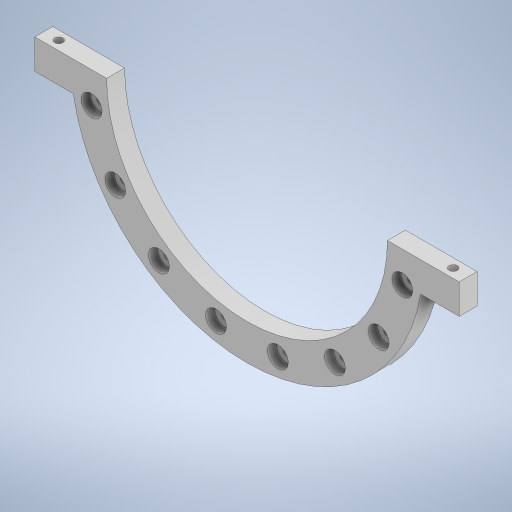
# Autodesk Inventor part: Постель 201 зад
Saved by Autodesk Inventor 2024.2 (Build 282272000, 272)
## iProperties
Created: 2024-04-28
Part Number: Постель 201 зад
Material: Generic
Document SubType Name: Sheet Metal
Designer: admin
Density: 1 g/cm^3
Appearance: Default
Stock Number: Постель_Корма
Flat Pattern Width: 29.5 cm
Flat Pattern Length: 71 cm
Flat Pattern Area: 2094.5 cm^2
Sheet Metal Rule: Default
Sheet Metal Width: 295,000 mm
Sheet Metal Length: 710,000 mm
Sheet Metal Area: 209450,000 mm^2
Author: pokla
Autodesk Inventor part; units mm, degrees
ref_plane "YZ Plane" through (0, 0, 0) normal (1, 0, 0) x (0, 1, 0)
ref_plane "XZ Plane" through (0, 0, 0) normal (0, 1, 0) x (-1, 0, 0)
ref_plane "XY Plane" through (0, 0, 0) normal (0, 0, 1) x (1, 0, 0)
sketch "Sketch1" plane through (0, 0, 0) normal (0, 0, 1) x (1, 0, 0)
  circle A0 centre (0, 0) radius 265 construction
  line L0 (0, 265) -> (0, 295) construction
  line L1 (0, 265) -> (0, 235) construction
  circle A1 centre (0, 0) radius 235
  circle A2 centre (0, 0) radius 295
  line L2 (-235, 0) -> (-235, 80) construction
  line L3 (-235, 80) -> (-295, 80) construction
  line L4 (-295, 80) -> (-295, 0) construction
  line L5 (235, 0) -> (235, 80) construction
  line L6 (235, 80) -> (295, 80) construction
  line L7 (295, 80) -> (295, 0) construction
  line L8 (-235, 0) -> (-295, 0)
  line L9 (-295, 0) -> (-355, 0)
  line L10 (-355, 0) -> (-355, -50)
  line L11 (-355, -50) -> (-290.7318, -50)
  line L12 (235, 0) -> (295, 0)
  line L13 (295, 0) -> (355, 0)
  line L14 (355, 0) -> (355, -50)
  line L15 (355, -50) -> (290.7318, -50)
  dimension "d13" = 530
  dimension "d26" = 80
  dimension "d36" = 60
  dimension "d40" = 60
  dimension "d41" = 50
  constraints: 32 end point, 8 point on circle, 7 perpendicular, 4 equal length, 4 horizontal, 4 tangent, 4 vertical, 3 coincident, 2 centre point, 1 line through centre, 1 point on line, 1 vertical alignment, 2 other
  measures "d26" distance of L2.start L2.end
  measures "d36" distance of L1.end L0.end
  measures "d40" distance of L4.end L9.end
  measures "d41" distance of L9.end L10.end
extrude "Extrusion1" add sketch "Sketch1" against normal blind 30 contours L12 A2 L8 A1 | L13 L14 L15 A2 | A2 L11 L10 L9 picked at (3.5144, -274.7637)
sketch "Sketch4" plane through (0, 0, 0) normal (0, 0, 1) x (1, 0, 0)
  line L0 (0, 0) -> (51.6989, -259.9081) construction
  line L1 (0, 0) -> (0, -276.8337) construction
  dimension "d27" = 265
  dimension "d35" = 11.25
  constraints: 4 end point, 1 coincident, 1 vertical
  measures "d27" distance of L0.end L0.start
  measures "d35" angle of L1 L0
sketch "Sketch7" plane through (0, 0, 0) normal (0, 0, 1) x (1, 0, 0)
  line L0 (-355, -50) -> (-355, 0) construction
  line L1 (-355, -25) -> (355, -25) construction
  line L2 (355, 0) -> (355, -50) construction
  point P0 (0, 0)
  point P1 (-330, -25)
  dimension "d42" = 25
  constraints: 2 end point, 2 midpoint, 1 point on line
  measures "d42" distance from line of point (-330, -25) L0
fillet "Fillet1" [suppressed]
hole "Hole1" [suppressed]
hole "Hole2" at (51.6989, -259.9081, 0) direction (0, 0, -1) diameter 13 end through all counterbore diameter 35 counterbore depth 15
pattern_circular "Circular Pattern4" count 9 over 180 about axis through (0, 0, -10) along (0, 0, -1) of "Hole2" both ways yes
mirror "Mirror1" [suppressed]
sketch "Sketch9" plane through (-355, 0, 0) normal (0, 1, 0) x (1, 0, 0)
  circle A0 centre (25, 15) radius 7
  line L0 (0, 0) -> (0, 30) projected
  point P0 (355, 0)
  point P1 (0, 15)
  dimension "d70" = 25
  dimension "d71" = 14
  constraints: 1 centre point, 1 horizontal alignment, 1 midpoint
  measures "d70" distance from line of L0 A0.centre
  measures "d71" diameter of A0
extrude "Extrusion8" cut sketch "Sketch9" against normal through all
mirror "Mirror2" about plane through (0, 0, 0) normal (1, 0, 0) of "Extrusion8"
equation "\"d13\" = Шпил_пласт_КОРМА_диам_центров"
equation "\"d40\" = d36"
equation "\"d27\" = 0.5 * Шпил_пласт_КОРМА_диам_центров"
equation "\"BendReliefDepth\" = 0.5 * Thickness"
equation "\"Шпил_пласт_КОРМА_диам_центров\" = 530"
equation "\"Thickness\" = 30"
body "Solid1"
